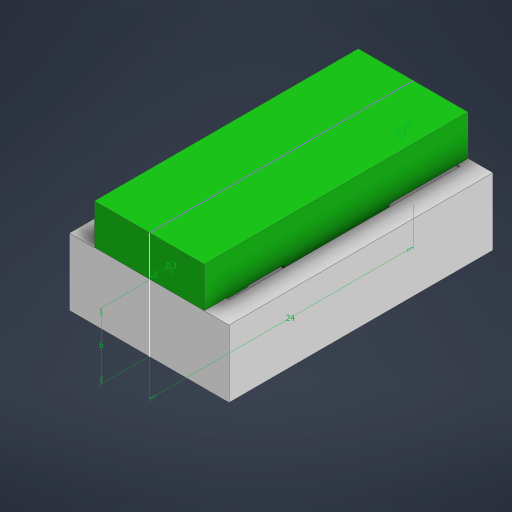
# Autodesk Inventor part: stanzev1u
Saved by Autodesk Inventor 2024.3 (Build 283343010, 343A)
## iProperties
Created: 2025-05-07
Part Number: stanzev1u
Material: Generisch
Document SubType Name: Modeling
Designer: David
Density: 1 g/cm^3
Appearance: Vorgabe
Author: David
## iProperties of the stored document stanzev1u_3D-Druck.ipt
Created: 2025-05-07
Part Number: stanzev1u_3D-Druck
Material: Generisch
Document SubType Name: Modeling
Designer: David
Density: 1 g/cm^3
Appearance: Vorgabe
Author: David
Autodesk Inventor part; units mm, degrees
ref_plane "YZ Plane" through (0, 0, 0) normal (1, 0, 0) x (0, 1, 0)
ref_plane "XZ Plane" through (0, 0, 0) normal (0, 1, 0) x (-1, 0, 0)
ref_plane "XY Plane" through (0, 0, 0) normal (0, 0, 1) x (1, 0, 0)
sketch "Skizze3" plane through (0, 0, 0) normal (1, 0, 0) x (0, 1, 0)
  line L0 (3, -0.1) -> (3, 0)
  line L1 (3, 0) -> (0, 0)
  line L2 (0, 0) -> (0, -0.1)
  line L3 (0, -0.1) -> (3, -0.1)
  line L4 (3, -0.1) -> (3, 0)
  arc A0 (3.1879, -0.2316) -> (3, -0.1) centre (3, -0.3) ccw
  line L5 (3.1879, -0.2316) -> (3.2819, -0.1974)
  arc A1 (3.2819, -0.1974) -> (3, 0) centre (3, -0.3) ccw
  line L6 (3.1879, -0.2316) -> (3.2819, -0.1974)
  line L7 (3.1879, -0.2316) -> (3.8565, -2.0684)
  line L8 (3.8565, -2.0684) -> (3.9505, -2.0342)
  line L9 (3.9505, -2.0342) -> (3.2819, -0.1974)
  line L10 (3.8565, -2.0684) -> (3.9505, -2.0342)
  arc A2 (3.8565, -2.0684) -> (4.0444, -2.2) centre (4.0444, -2) ccw
  line L11 (4.0444, -2.2) -> (4.0444, -2.1)
  arc A3 (3.9505, -2.0342) -> (4.0444, -2.1) centre (4.0444, -2) ccw
  line L12 (4.0444, -2.2) -> (11.9556, -2.2)
  line L13 (4.0444, -2.2) -> (4.0444, -2.1)
  line L14 (4.0444, -2.2) -> (11.9556, -2.2)
  line L15 (11.9556, -2.2) -> (11.9556, -2.1)
  line L16 (11.9556, -2.1) -> (4.0444, -2.1)
  line L17 (11.9556, -2.2) -> (11.9556, -2.1)
  arc A4 (11.9556, -2.2) -> (12.1435, -2.0684) centre (11.9556, -2) ccw
  line L18 (12.1435, -2.0684) -> (12.0495, -2.0342)
  arc A5 (11.9556, -2.1) -> (12.0495, -2.0342) centre (11.9556, -2) ccw
  line L19 (12.1435, -2.0684) -> (12.0495, -2.0342)
  line L20 (12.1435, -2.0684) -> (12.8121, -0.2316)
  line L21 (12.8121, -0.2316) -> (12.7181, -0.1974)
  line L22 (12.7181, -0.1974) -> (12.0495, -2.0342)
  line L23 (12.8121, -0.2316) -> (12.7181, -0.1974)
  arc A6 (13, -0.1) -> (12.8121, -0.2316) centre (13, -0.3) ccw
  line L24 (13, -0.1) -> (13, 0)
  arc A7 (13, 0) -> (12.7181, -0.1974) centre (13, -0.3) ccw
  line L25 (13, -0.1) -> (13, 0)
  line L26 (13, -0.1) -> (16, -0.1)
  line L27 (16, 0) -> (16, -0.1)
  line L28 (16, 0) -> (13, 0)
  line L29 (0, -0.1) -> (-4, -0.1)
  line L30 (-4, -0.1) -> (-4, -6.1)
  line L31 (-4, -6.1) -> (20, -6.1)
  line L32 (20, -6.1) -> (20, -0.1)
  line L33 (16, -0.1) -> (20, -0.1)
  line L34 (-4, 0) -> (-2, 0)
  line L35 (-2, 0) -> (-2, -0.1)
  line L36 (-2, -0.1) -> (-4, -0.1)
  line L37 (-4, -0.1) -> (-4, 0)
  line L38 (19, -0.1) -> (20, -0.1)
  line L39 (20, -0.1) -> (20, 0)
  line L40 (20, 0) -> (19, 0)
  line L41 (19, 0) -> (19, -0.1)
  line L42 (20, 0) -> (20, 3.6516)
  line L43 (20, 3.6516) -> (-4, 3.6516)
  line L44 (-4, 3.6516) -> (-4, -0.1)
  line L45 (16, 0) -> (19, 0)
  point P0 (16, -0.1)
  point P1 (8, -6.1)
  point P2 (8, -2.1)
  dimension "d13" = 24
  dimension "d14" = 6
  dimension "d17" = 2
  dimension "d18" = 0.1
  dimension "d19" = 1
  dimension "d20" = 0.1
  constraints: 92 end point, 16 point on circle, 11 horizontal, 11 vertical, 8 centre point, 5 parallel, 5 perpendicular, 3 midpoint, 3 point on line, 1 vertical alignment, 67 other
  measures "d13" distance of L30.end L31.end
  measures "d14" distance of L29.end L30.end
  measures "d17" distance of L34.start L34.end
  measures "d18" distance of L34.end L35.end
  measures "d19" distance of L39.end L40.end
  measures "d20" distance of L40.end L38.start
extrude "Extrusion2" add sketch "Skizze3" along normal mid plane 10.5 contours A0 L7 A2 L12 A4 L20 A6 L26 L33 L32 L31 L30 L29 L3 | L29 L37 L34 L35 | L33 L41 L40 L39 | L21 A7 L24 A6
sketch "Skizze4" plane through (-5.25, -4, -6.1) normal (0, -1, 0) x (1, 0, 0)
  line L0 (10.5, 6.1) -> (10.5, 0) projected
  line L1 (10.5, 6.1) -> (12.5, 6.1)
  line L2 (12.5, 6.1) -> (12.5, 0)
  line L3 (12.5, 0) -> (10.5, 0)
  line L4 (10.5, 0) -> (10.5, 6.1)
  line L5 (0, 6.1) -> (-2, 6.1)
  line L6 (-2, 6.1) -> (-2, 0)
  line L7 (-2, 0) -> (0, 0)
  line L8 (0, 0) -> (0, 6.1)
  point P0 (5.25, 6.1)
  dimension "d24" = 2
  dimension "d31" = 2
  constraints: 16 end point, 4 parallel, 2 horizontal, 2 perpendicular
  measures "d24" distance of L0.start L1.end
  measures "d31" distance of L5.start L5.end
extrude "Extrusion3" add sketch "Skizze4" against normal up to surface (24 mm away)
extrude "Extrusion4" add sketch "Skizze3" along normal mid plane 10 separate body contours L1 L2 L29 L35 L34 L44 L43 L42 L40 L45 L28 A7 L22 A5 L16 A3 L9 A1
